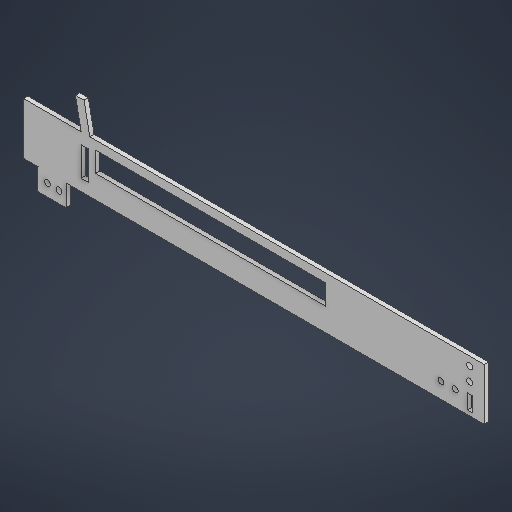
# Autodesk Inventor part: Middle_bar
Saved by Autodesk Inventor 2027 (Build 310192000, 192)
## iProperties
Created: 2026-05-09
Part Number: Middle_bar
Material: Generic
Document SubType Name: Modeling
Designer: alexy
Density: 1 g/cm^3
Appearance: Default
Mass: 26.8499 g
Surface Area: 216.911 cm^2
Volume: 26.8499 cm^3
Author: alexy
Autodesk Inventor part; units mm, degrees
ref_plane "YZ Plane" through (0, 0, 0) normal (1, 0, 0) x (0, 1, 0)
ref_plane "XZ Plane" through (0, 0, 0) normal (0, 1, 0) x (-1, 0, 0)
ref_plane "XY Plane" through (0, 0, 0) normal (0, 0, 1) x (1, 0, 0)
sketch "Sketch1" plane through (0, 0, 0) normal (0, 0, 1) x (1, 0, 0)
  line L0 (0, 0) -> (320, 0)
  line L1 (320, 0) -> (320, 16)
  line L2 (320, 16) -> (0, 16)
  line L3 (0, 16) -> (0, 0)
  line L4 (0, 0) -> (22.0483, 0)
  line L5 (10, 0) -> (29.5, 0)
  line L6 (29.5, 0) -> (29.5, -15)
  line L7 (29.5, -15) -> (10, -15)
  line L8 (10, -15) -> (10, 0)
  line L9 (308.4, 13.1) -> (311.6, 13.1)
  line L10 (311.6, 13.1) -> (311.6, 2.9)
  line L11 (311.6, 2.9) -> (308.4, 2.9)
  line L12 (308.4, 2.9) -> (308.4, 13.1)
  line L13 (308.4, 13.1) -> (311.6, 2.9) construction
  line L14 (311.6, 13.1) -> (308.4, 2.9) construction
  circle A0 centre (300, 11) radius 2.05
  circle A1 centre (290, 11) radius 2.05
  point P0 (0, 8)
  point P1 (310, 8)
  dimension "d2" = 19.5
  dimension "d3" = 15
  dimension "d4" = 10
  dimension "d5" = 16
  dimension "d8" = 320
  dimension "d13" = 10.2
  dimension "d14" = 3.2
  dimension "d15" = 10
  dimension "d16" = 4.1
  dimension "d18" = 4.1
  dimension "d20" = 10
  dimension "d21" = 20
  dimension "d23" = 5
  constraints: 30 end point, 6 parallel, 4 horizontal, 3 midpoint, 3 perpendicular, 2 centre point, 2 horizontal alignment, 1 point on line
  measures "d2" distance of L6.end L7.end
  measures "d3" distance of L5.end L6.end
  measures "d4" distance of L0.start L5.start
  measures "d5" distance of L2.end L0.start
  measures "d8" distance of L1.end L2.end
  measures "d13" distance of L10.start L10.end
  measures "d14" distance of L10.end L11.end
  measures "d15" distance from line of L1 point (310, 8)
  measures "d16" diameter of A0
  measures "d18" diameter of A1
  measures "d20" distance of A1.centre A0.centre
  measures "d21" distance from line of L1 A0.centre
  measures "d23" distance from line of L2 A1.centre
extrude "Extrusion1" add sketch "Sketch1" along normal blind 3
sketch "Sketch2" plane through (0, 0, 3) normal (0, 0, 1) x (1, 0, 0)
  line L0 (0, 16) -> (0, 0) projected
  line L1 (0, 16) -> (0, 36)
  line L2 (320, 0) -> (320, 16) projected
  line L3 (320, 16) -> (320, 36)
  line L4 (320, 36) -> (0, 36)
  line L5 (320, 16) -> (0, 16) projected
  line L6 (50, 16) -> (50, 30)
  line L7 (50, 30) -> (210, 30)
  line L8 (210, 30) -> (210, 16)
  line L9 (40, 36) -> (36, 56)
  line L10 (36, 56) -> (42, 56)
  line L11 (42, 56) -> (46, 36)
  circle A0 centre (300, 11) radius 2.05 projected
  line L12 (311.6, 13.1) -> (311.6, 2.9) projected
  circle A1 centre (310, 30) radius 2.1
  circle A2 centre (310, 20.6) radius 2.1
  point P0 (308.4, 13.1)
  point P1 (311.6, 8)
  dimension "d44" = 20
  dimension "d45" = 160
  dimension "d46" = 50
  dimension "d47" = 14
  dimension "d48" = 20
  dimension "d49" = 6
  dimension "d50" = 4
  dimension "d51" = 40
  dimension "d83" = 4.2
  dimension "d84" = 4.2
  dimension "d85" = 6
  dimension "d86" = 9.4
  dimension "d87" = 10
  constraints: 18 end point, 4 perpendicular, 4 point on line, 2 centre point, 2 parallel, 2 vertical, 1 midpoint, 1 vertical alignment
  measures "d44" distance of L0.start L1.end
  measures "d45" distance of L6.end L7.end
  measures "d46" distance between parallel lines of L1 L6
  measures "d47" distance of L6.start L6.end
  measures "d48" distance between parallel lines of L4 L10
  measures "d49" distance of L9.end L10.end
  measures "d50" horizontal distance of L9.start L9.end
  measures "d51" distance of L1.end L9.start
  measures "d83" diameter of A1
  measures "d84" diameter of A2
  measures "d85" distance from line of L4 A1.centre
  measures "d86" distance of A2.centre A1.centre
  measures "d87" distance from line of L3 A1.centre
extrude "Extrusion2" add sketch "Sketch2" against normal blind 3 contours L1 L4 L3 L5 L8 L7 L6 | L9 L10 L11 L4
sketch "Sketch3" plane through (0, 0, 3) normal (0, 0, 1) x (1, 0, 0)
  circle A0 centre (16.5, -6.5) radius 2.1
  circle A1 centre (24.5, -7) radius 2.1
  line L0 (29.5, 0) -> (320, 0) projected
  line L1 (29.5, -15) -> (29.5, 0) projected
  point P0 (0, 0)
  dimension "d75" = 4.2
  dimension "d76" = 6.5
  dimension "d77" = 4.2
  dimension "d78" = 7
  dimension "d79" = 5
  dimension "d80" = 8
  constraints: 2 centre point
  measures "d75" diameter of A0
  measures "d76" vertical distance of point (0, 0) A0.centre
  measures "d77" diameter of A1
  measures "d78" distance from line of L0 A1.centre
  measures "d79" distance from line of L1 A1.centre
  measures "d80" horizontal distance of A1.centre A0.centre
extrude "Extrusion3" cut sketch "Sketch3" against normal blind 3
sketch "Sketch4" plane through (0, 0, 3) normal (0, 0, 1) x (1, 0, 0)
  line L0 (39.9, 28.2) -> (45, 28.2)
  line L1 (45, 28.2) -> (45, 8)
  line L2 (45, 8) -> (39.9, 8)
  line L3 (39.9, 8) -> (39.9, 28.2)
  line L4 (50, 16) -> (50, 30) projected
  line L5 (29.5, 0) -> (320, 0) projected
  point P0 (0, 0)
  dimension "d88" = 5.1
  dimension "d89" = 20.2
  dimension "d90" = 5
  dimension "d91" = 8
  constraints: 8 end point, 2 parallel, 1 horizontal, 1 perpendicular
  measures "d88" distance of L1.end L2.end
  measures "d89" distance of L0.end L1.end
  measures "d90" distance between parallel lines of L4 L1
  measures "d91" distance between parallel lines of L5 L2
extrude "Extrusion4" cut sketch "Sketch4" against normal blind 3
body "Solid1"
